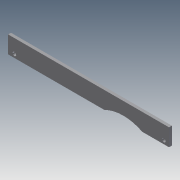
# Autodesk Inventor part: small
Saved by Autodesk Inventor 2011 (Build 150239000, 239)
## iProperties
Created: 2011-12-18
Part Number: small
Document SubType Name: Modeling
Designer: Matthew
Density: 1 g/cm^3
Author: Matthew
Autodesk Inventor part; units mm, degrees
ref_plane "YZ Plane" through (0, 0, 0) normal (1, 0, 0) x (0, 1, 0)
ref_plane "XZ Plane" through (0, 0, 0) normal (0, 1, 0) x (-1, 0, 0)
ref_plane "XY Plane" through (0, 0, 0) normal (0, 0, 1) x (1, 0, 0)
sketch "Sketch1" plane through (0, 0, 0) normal (0, 0, 1) x (1, 0, 0)
  line L0 (-27.2578, 3.3251) -> (156.8922, 3.3251)
  line L1 (156.8922, 3.3251) -> (156.8922, -9.3749)
  line L2 (156.8922, -9.3749) -> (-27.2578, -9.3749)
  line L3 (-27.2578, -9.3749) -> (-27.2578, 3.3251)
  line L4 (64.8172, -3.0249) -> (-20.7173, -3.0249)
  line L5 (-20.7173, -3.0249) -> (150.3517, -3.0249)
  line L6 (-20.7173, -3.0249) -> (-20.7173, -5.5649)
  circle A0 centre (-20.7173, -5.5649) radius 1.9812
  circle A1 centre (150.3517, -5.5649) radius 1.9812
  point P0 (0, 0)
  dimension "d0" = 184.15
  dimension "d1" = 12.7
  dimension "d2" = 85.5345
  dimension "d3" = 171.069
  dimension "d4" = 2.54
  dimension "d5" = 3.9624
  constraints: 14 end point, 3 parallel, 3 perpendicular, 2 centre point, 1 coincident, 1 horizontal
  measures "d0" distance of L1.end L2.end
  measures "d1" distance of L0.end L1.end
  measures "d2" distance of L4.start L4.end
  measures "d3" distance of L4.end L5.end
  measures "d4" distance of L4.end L6.end
  measures "d5" diameter of A0
extrude "Extrusion1" add sketch "Sketch1" along normal blind 3.175
sketch "Sketch2" plane through (-27.2578, 3.3251, 0) normal (0, 1, 0) x (1, 0, 0)
  line L0 (0, -3.175) -> (184.15, -3.175) projected
  line L1 (184.15, 0) -> (184.15, -3.175) projected
  line L2 (0, 0) -> (184.15, 0) projected
  line L3 (0, 0) -> (0, -3.175) projected
  point P0 (27.2578, 0)
extrude "Extrusion2" add sketch "Sketch2" along normal blind 6.35
sketch "Sketch3" plane through (0, 0, 3.175) normal (0, 0, 1) x (1, 0, 0)
  circle A0 centre (150.3517, -5.5649) radius 1.9812 projected
  circle A1 centre (-20.7173, -5.5649) radius 1.9812 projected
  point P0 (0, 0)
extrude "Extrusion3" add sketch "Sketch3" against normal blind 6.35
sketch "Sketch4" plane through (0, 0, 3.175) normal (0, 0, 1) x (1, 0, 0)
  line L0 (156.8922, -9.3749) -> (-27.2578, -9.3749) projected
  line L1 (64.8172, -9.3749) -> (64.8172, -5.5649)
  line L2 (64.8172, -5.5649) -> (-17.7328, -5.5649)
  circle A0 centre (-17.7328, -5.5649) radius 1.9812
  line L3 (-17.7328, -5.5649) -> (147.3672, -5.5649)
  circle A1 centre (147.3672, -5.5649) radius 1.9812
  point P0 (0, 0)
  dimension "d12" = 3.81
  dimension "d13" = 82.55
  dimension "d14" = 3.9624
  dimension "d15" = 165.1
  constraints: 6 end point, 2 centre point, 2 coincident, 2 perpendicular, 1 midpoint, 1 point on line
  measures "d12" distance of L1.start L1.end
  measures "d13" distance of L1.end L2.end
  measures "d14" diameter of A0
  measures "d15" distance of L3.start L3.end
extrude "Extrusion4" cut sketch "Sketch4" against normal blind 6.35
sketch "Sketch5" plane through (156.8922, -9.3749, 3.175) normal (1, 0, 0) x (0, 0, -1)
  line L0 (0, 19.05) -> (0, 0) projected
  line L1 (3.175, 0) -> (0, 0) projected
  line L2 (3.175, 19.05) -> (3.175, 0) projected
  line L3 (3.175, 19.05) -> (0, 19.05) projected
  point P0 (3.175, 9.3749)
extrude "Extrusion5" cut sketch "Sketch5" against normal blind 3.81
sketch "Sketch6" plane through (-27.2578, -9.3749, 0) normal (-1, 0, 0) x (0, 0, 1)
  line L0 (3.175, 0) -> (3.175, 19.05) projected
  line L1 (3.175, 19.05) -> (0, 19.05) projected
  line L2 (0, 0) -> (0, 19.05) projected
  line L3 (0, 0) -> (3.175, 0) projected
  point P0 (0, 9.3749)
extrude "Extrusion6" cut sketch "Sketch6" against normal blind 2.54
sketch "Sketch7" plane through (0, 0, -3.175) normal (0, 0, -1) x (-1, 0, 0)
  arc A0 (-148.8595, -4.2617) -> (-148.8595, -6.8681) centre (-147.3672, -5.5649) ccw projected
  arc A1 (-148.8595, -4.2617) -> (-148.8595, -6.8681) centre (-150.3517, -5.5649) ccw projected
  point P0 (0, 0)
extrude "Extrusion7" cut sketch "Sketch7" against normal blind 3.175
sketch "Sketch8" plane through (0, 0, -3.175) normal (0, 0, -1) x (-1, 0, 0)
  arc A0 (19.225, -6.8681) -> (19.225, -4.2617) centre (17.7328, -5.5649) ccw projected
  arc A1 (19.225, -6.8681) -> (19.225, -4.2617) centre (20.7173, -5.5649) ccw projected
  point P0 (0, 0)
extrude "Extrusion8" cut sketch "Sketch8" against normal blind 3.175
sketch "Sketch9" plane through (0, 0, 0) normal (0, 0, -1) x (-1, 0, 0)
  line L0 (-153.0822, -9.3749) -> (24.7178, -9.3749) projected
  circle A0 centre (-147.3672, -5.5649) radius 1.9812 projected
  line L1 (-147.3672, -5.5649) -> (-102.5362, -5.5649)
  line L2 (-102.5362, -5.5649) -> (-102.5362, -50.3959)
  circle A1 centre (-102.5362, -50.3959) radius 46.0375
  point P0 (0, 0)
  dimension "d26" = 44.831
  dimension "d27" = 44.831
  dimension "d28" = 92.075
  constraints: 4 end point, 1 centre point, 1 coincident, 1 parallel, 1 perpendicular
  measures "d26" distance of L1.start L1.end
  measures "d27" distance of L1.end L2.end
  measures "d28" diameter of A1
extrude "Extrusion9" cut sketch "Sketch9" against normal blind 25.4 contours A1 L1 L2 L0 | L0 A1 | L2 L1 A1 L0
body "Solid1"
